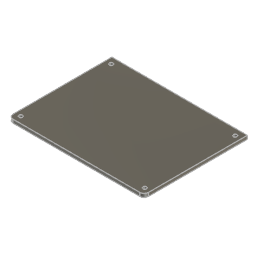
PCB Base (Autodesk Fusion 360 design; units mm, degrees)
part number: 2026-07-11-17-10-09-856
Autodesk Fusion 360 part; units mm, degrees
sketch "Sketch1" plane through (0, 0, 0) normal (0, 0, 1) x (1, 0, 0)
  line L0 (-47.25, 36) -> (47.25, 36)
  line L1 (47.25, 36) -> (47.25, -36)
  line L2 (47.25, -36) -> (-47.25, -36)
  line L3 (-47.25, -36) -> (-47.25, 36)
  line L4 (-47.25, 36) -> (47.25, -36) construction
  line L5 (47.25, 36) -> (-47.25, -36) construction
  circle A0 centre (-43.25, 31.5) radius 1.25
  circle A1 centre (-43.25, -31.5) radius 1.25
  circle A2 centre (43.25, 31.5) radius 1.25
  circle A3 centre (43.25, -31.5) radius 1.25
  dimension "d1" = 94.5
  dimension "d2" = 72
  dimension "d3" = 2.5
  dimension "d4" = 86.5
  dimension "d5" = 63
  dimension "d6" = 31.5
  dimension "d7" = 43.25
  constraint horizontal L0
  constraint perpendicular L0 L1
  constraint parallel L0 L2
  constraint parallel L1 L3
  constraint coincident L4 origin
  constraint coincident L5 origin
  constraint vertical A0.centre A1.centre
  constraint horizontal A1.centre A3.centre
  constraint vertical A2.centre A3.centre
  constraint horizontal A0.centre A2.centre
  constraint equal A1 A2
  constraint equal A2 A3
  constraint equal A0 A3
  measures "d1" distance of L0.start L0.end
  measures "d2" distance of L0.start L2.end
  measures "d3" diameter of A0
  measures "d4" distance of A0.centre A2.centre
  measures "d5" distance of A0.centre A1.centre
  measures "d6" vertical distance of origin A1.centre
  measures "d7" horizontal distance of origin A0.centre
extrude "Extrude1" add sketch "Sketch1" along normal blind 2.5
fillet "Fillet1" radius 3 2 edges at (47.25, -36, 1.25) (-47.25, -36, 1.25)
sketch "Sketch2" plane through (0, 0, 2.5) normal (0, 0, 1) x (-1, 0, 0)
  arc A0 (47.25, 33) -> (44.25, 36) centre (44.25, 33) ccw
  line L0 (44.25, 36) -> (-44.25, 36)
  arc A1 (-44.25, 36) -> (-47.25, 33) centre (-44.25, 33) ccw
  line L1 (-47.25, 33) -> (-47.25, -36)
  line L2 (-47.25, -36) -> (47.25, -36)
  line L3 (47.25, -36) -> (47.25, 33)
  circle A2 centre (-43.25, -31.5) radius 1.25
  circle A3 centre (43.25, -31.5) radius 1.25
  circle A4 centre (43.25, 31.5) radius 1.25
  circle A5 centre (-43.25, 31.5) radius 1.25
  circle A6 centre (43.25, 31.5) radius 1.5
  constraint concentric A4 A6
equation "d1 = 90.5 mm + 4 mm"
equation "d2 = 67 mm + 5 mm"
equation "d6 = ( d5 / 2 mm ) * 1 mm"
equation "d7 = d4 / 2"
